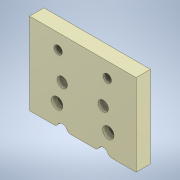
# Autodesk Inventor part: Soporte Extruder Izq
Saved by Autodesk Inventor 2021 (Build 250183000, 183)
## iProperties
Created: 2023-01-29
Part Number: Soporte Extruder Izq
Material: Polipropileno
Document SubType Name: Modeling
Designer: Diego.labarca
Density: 0.899 g/cm^3
Appearance: Suave - Fresno
Mass: 57.1428 g
Surface Area: 54.9661 cm^2
Volume: 12.6702 cm^3
Author: Diego.labarca
Autodesk Inventor part; units mm, degrees
ref_plane "YZ Plane" through (0, 0, 0) normal (1, 0, 0) x (0, 1, 0)
ref_plane "XZ Plane" through (0, 0, 0) normal (0, 1, 0) x (-1, 0, 0)
ref_plane "XY Plane" through (0, 0, 0) normal (0, 0, 1) x (1, 0, 0)
sketch "Boceto21" plane through (0, 0, 0) normal (0, 0, 1) x (1, 0, 0)
  line L0 (-26, 15) -> (26, 15)
  line L1 (26, 15) -> (26, -15)
  line L2 (26, -15) -> (-26, -15)
  line L3 (-26, -15) -> (-26, 15)
  line L4 (1.8793, 0) -> (0, 0)
  line L5 (0, 0) -> (0, 2.1218)
  dimension "d96" = 52
  dimension "d97" = 30
  constraints: 12 end point, 2 horizontal, 2 parallel, 2 perpendicular, 2 other
  measures "d96" distance of L1.end L2.end
  measures "d97" distance of L0.end L1.end
extrude "Extrusión17" add sketch "Boceto21" along normal blind 7
sketch "Boceto22" plane through (0, 0, 7) normal (0, 0, 1) x (1, 0, 0)
  circle A0 centre (-12.5, -5) radius 1.5
  circle A1 centre (12.5, -5) radius 1.5
  line L0 (-26, -15) -> (26, -15) projected
  point P0 (0, 0)
  dimension "d100" = 3
  dimension "d101" = 3
  dimension "d104" = 10
  dimension "d105" = 10
  dimension "d106" = 25
  dimension "d107" = 12.5
  constraints: 2 centre point
  measures "d100" diameter of A0
  measures "d101" diameter of A1
  measures "d104" distance from line of L0 A0.centre
  measures "d105" distance from line of L0 A1.centre
  measures "d106" distance of A0.centre A1.centre
  measures "d107" horizontal distance of A0.centre point (0, 0)
extrude "Extrusión18" cut sketch "Boceto22" against normal through all
sketch "Boceto23" plane through (0, 0, 7) normal (0, 0, 1) x (1, 0, 0)
  circle A0 centre (10, 5) radius 2.5
  circle A1 centre (10, -15) radius 2.5
  circle A2 centre (12.5, -5) radius 1.5 projected
  point P0 (0, 0)
  dimension "d110" = 5
  dimension "d111" = 5
  dimension "d112" = 10
  dimension "d113" = 10
  dimension "d114" = 20
  dimension "d115" = 10
  constraints: 2 centre point
  measures "d110" diameter of A0
  measures "d111" diameter of A1
  measures "d112" horizontal distance of point (0, 0) A1.centre
  measures "d113" horizontal distance of point (0, 0) A0.centre
  measures "d114" distance of A1.centre A0.centre
  measures "d115" vertical distance of A1.centre A2.centre
extrude "Extrusión19" cut sketch "Boceto23" against normal through all contours A0 | A1
mirror "Simetría1" about plane through (0, 0, 0) normal (1, 0, 0) of "Extrusión19"
fillet "Empalme5" radius 2 4 edges at (-12.5, -15, 3.5) (-7.5, -15, 3.5) (12.5, -15, 3.5) (7.5, -15, 3.5)
sketch "Boceto24" plane through (0, 0, 7) normal (0, 0, 1) x (1, 0, 0)
  circle A0 centre (12.5, -5) radius 1.5 projected
  circle A1 centre (12.5, -5) radius 2.75
  circle A2 centre (-12.5, -5) radius 1.5 projected
  circle A3 centre (-12.5, -5) radius 2.75
  point P0 (0, 0)
  dimension "d119" = 5.5
  dimension "d120" = 5.5
  constraints: 2 centre point, 2 coincident
  measures "d119" diameter of A1
  measures "d120" diameter of A3
extrude "Extrusión20" cut sketch "Boceto24" against normal blind 3
sketch "Boceto25" plane through (0, 0, 7) normal (0, 0, 1) x (1, 0, 0)
  line L0 (26, 15) -> (-26, 15)
  line L1 (-26, 15) -> (-26, 25)
  line L2 (-26, 25) -> (26, 25)
  line L3 (26, 25) -> (26, 15)
  point P0 (0, 0)
  dimension "d123" = 10
  constraints: 8 end point, 2 parallel, 1 horizontal, 1 perpendicular
  measures "d123" distance of L0.end L1.end
extrude "Extrusión21" add sketch "Boceto25" against normal up to surface (7 mm away)
sketch "Boceto26" plane through (0, 0, 7) normal (0, 0, 1) x (1, 0, 0)
  circle A0 centre (12, 17.682) radius 2
  circle A1 centre (12.5, -5) radius 2.75 projected
  circle A2 centre (-12, 17.682) radius 2
  circle A3 centre (-12.5, -5) radius 2.75 projected
  circle A4 centre (10, 5) radius 2.5 projected
  circle A5 centre (-10, 5) radius 2.5 projected
  point P0 (0, 0)
  dimension "d127" = 12
  dimension "d128" = 4
  dimension "d129" = 4
  dimension "d132" = 12
  dimension "d135" = 12.682
  dimension "d136" = 12.682
  constraints: 2 centre point
  measures "d127" horizontal distance of point (0, 0) A0.centre
  measures "d128" diameter of A2
  measures "d129" diameter of A0
  measures "d132" horizontal distance of point (0, 0) A2.centre
  measures "d135" vertical distance of A4.centre A0.centre
  measures "d136" vertical distance of A5.centre A2.centre
extrude "Extrusión22" cut sketch "Boceto26" against normal through all contours A0 | A2
equation "\"d101\" = d100"
equation "\"d105\" = d104"
equation "\"d107\" = 0.5 * d106"
equation "\"d111\" = d110"
equation "\"d113\" = d112"
equation "\"d120\" = d119"
equation "\"d128\" = d129"
equation "\"d136\" = d135"
